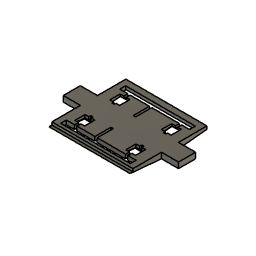
battery mount top v9 (Autodesk Fusion 360 design; units mm, degrees)
Autodesk Fusion 360 part; units mm, degrees
note: some values were not read from the file. Set by a fixed rule: which face or edge a step refers to.
sketch "Sketch1" plane through (0, 0, 0) normal (0, 0, 1) x (1, 0, 0)
  line L0 (0, 0) -> (180.975, 0)
  line L1 (0, 0) -> (0, -165.1)
  line L2 (0, -165.1) -> (180.975, -165.1)
  line L3 (180.975, 0) -> (180.975, -165.1)
  dimension "d1" = 180.975
  dimension "d2" = 180.975
  dimension "d36" = 165.1
  constraint coincident L0.start L1.start
  constraint horizontal L0
  constraint perpendicular L0 L1
  constraint perpendicular L1 L2
  measures "d1" distance of L0.start L0.end
  measures "d2" distance of L1.end L2.end
  measures "d36" distance of L0 L2
extrude "Extrude1" add sketch "Sketch1" along normal blind 6.35
sketch "Sketch2" plane through (0, 0, 6.35) normal (0, 0, 1) x (-1, 0, 0)
  line L0 (0, 0) -> (0, 165.1)
  line L1 (0, 165.1) -> (-180.975, 165.1)
  line L2 (-180.975, 165.1) -> (-180.975, 0)
  line L3 (-180.975, 0) -> (0, 0)
sketch "Sketch4" plane through (0, 0, 0) normal (0, 0, -1) x (1, 0, 0)
  line L0 (0, 165.1) -> (0, 0)
  line L1 (0, 0) -> (180.975, 0)
  line L2 (180.975, 0) -> (180.975, 165.1)
  line L3 (180.975, 165.1) -> (0, 165.1)
  line L4 (193.675, 57.15) -> (0, 57.15)
  line L5 (0, 107.95) -> (193.675, 107.95)
  line L6 (180.975, 0, -6.35) -> (0, 0, -6.35)
  line L7 (0, 165.1, -6.35) -> (180.975, 165.1, -6.35)
  line L8 (193.675, 107.95) -> (193.675, 57.15)
  dimension "d33" = 50.8
  dimension "d34" = 57.15
  dimension "d41" = 193.675
  constraint coincident L0 L4.end
  constraint perpendicular L0 L4
  constraint coincident L0 L5.start
  constraint perpendicular L2 L5
  measures "d33" distance of L4 L5
  measures "d34" distance of L1 L4
  measures "d41" distance of L5.start L5.end
sketch "Sketch5" plane through (0, 0, 0) normal (1, 0, 0) x (0, 1, 0)
  line L0 (-69.85, -6.35) -> (0, 0)
  line L1 (-95.2638, -6.3731) -> (-165.1, 0)
  line L2 (-69.85, -6.35) -> (-69.85, 0)
  line L3 (-69.85, 0) -> (0, 0)
  line L4 (-95.2638, -6.3731) -> (-95.2638, 0)
  line L5 (-95.2638, 0) -> (-165.1, 0)
  constraint coincident L0.end L3.end
  constraint vertical L2
  constraint perpendicular L2 L3
  constraint perpendicular L3 L4
  constraint perpendicular L4 L5
sketch "Sketch10" plane through (0, 0, 0) normal (-1, 0, 0) x (0, -1, 0)
  line L0 (0, 0) -> (165.1, 0)
  line L1 (165.1, 0) -> (165.1, 6.35)
  line L2 (165.1, 6.35) -> (0, 6.35)
  line L3 (0, 6.35) -> (0, 0)
  line L4 (165.1, 0) -> (69.85, 0)
  line L5 (69.85, 0) -> (69.85, -6.35)
  constraint coincident L0.end L1.start
sketch "Sketch11" plane through (0, 0, 0) normal (0, 0, -1) x (1, 0, 0)
  line L0 (0, 165.1) -> (0, 0)
  line L1 (0, 0) -> (180.975, 0)
  line L2 (180.975, 0) -> (180.975, 165.1)
  line L3 (180.975, 165.1) -> (0, 165.1)
  line L4 (-38.1, 101.6) -> (219.075, 101.6)
  line L5 (219.075, 101.6) -> (219.075, 63.5)
  line L6 (219.075, 63.5) -> (-38.1, 63.5)
  line L7 (-38.1, 63.5) -> (-38.1, 101.6)
  dimension "d67" = 38.1
  dimension "d68" = 38.1
  dimension "d69" = 38.1
  dimension "d70" = 63.5
  dimension "d71" = 165.1
  constraint horizontal L4
  constraint vertical L5
  constraint horizontal L6
  constraint vertical L7
  measures "d67" distance of L0 L7
  measures "d68" distance of L2 L5
  measures "d69" distance of L4 L6
  measures "d70" distance of L3 L4
  measures "d71" distance of L0.start L0.end
extrude "Extrude12" add sketch "Sketch11" along normal blind 6.35 and the other way blind 6.35 contours L0 L2 L4 L6 | L0 L4 L6 L7 | L2 L4 L5 L6
sketch "Sketch12" plane through (0, 0, 0) normal (1, 0, 0) x (0, 1, 0)
  line L0 (-101.6, -6.35) -> (-171.4692, 0)
  line L1 (-171.4692, 0) -> (-101.6, 0)
  line L2 (-101.6, 0) -> (-101.6, -6.35)
  line L3 (-63.5, -6.35) -> (0, 0)
  line L4 (0, 0) -> (-63.5, 0)
  line L5 (-63.5, 0) -> (-63.5, -6.35)
  line L6 (-101.6, -6.35, 219.075) -> (-101.6, -6.35, -38.1)
  line L7 (-63.5, -6.35, -38.1) -> (-63.5, -6.35, 219.075)
  point P0 (-63.5, 0)
  constraint horizontal L1
  constraint perpendicular L1 L2
  constraint coincident L3.end L4.start
  constraint perpendicular L2 L4
  constraint parallel L2 L5
  constraint coincident P0 L4.end
extrude "Extrude13" add sketch "Sketch12" along normal up to surface (180.975 mm away)
sketch "Sketch13" plane through (0, -1.4047, -15.4562) normal (0, -0.090511, -0.995895) x (1, 0, 0)
  line L0 (180.975, 100.6082) -> (180.975, 170.7654)
  line L1 (0, 170.7654) -> (0, 100.6082)
  line L2 (180.975, 170.7654) -> (0, 170.7654)
  line L3 (-89.535, 82.5409) -> (270.51, 82.5409)
  line L4 (161.925, 110.2854) -> (131.925, 110.2854)
  line L5 (131.925, 110.2854) -> (131.925, 140.2854)
  line L6 (131.925, 140.2854) -> (161.925, 140.2854)
  line L7 (161.925, 140.2854) -> (161.925, 110.2854)
  line L8 (12.7, 158.0654) -> (168.275, 158.0654)
  line L9 (168.275, 158.0654) -> (168.275, 145.3654)
  line L10 (168.275, 145.3654) -> (12.7, 145.3654)
  line L11 (12.7, 145.3654) -> (12.7, 158.0654)
  line L12 (49.05, 140.2854) -> (49.05, 110.2854)
  line L13 (19.05, 140.2854) -> (49.05, 140.2854)
  line L14 (19.05, 110.2854) -> (19.05, 140.2854)
  line L15 (49.05, 110.2854) -> (19.05, 110.2854)
  line L16 (81.4496, 145.3654) -> (76.3696, 145.3654)
  line L17 (76.3696, 145.3654) -> (76.3696, 109.8054)
  line L18 (76.3696, 109.8054) -> (81.4496, 109.8054)
  line L19 (81.4496, 109.8054) -> (81.4496, 145.3654)
  line L20 (36.2004, 145.3654) -> (31.1204, 145.3654)
  line L21 (31.1204, 145.3654) -> (31.1204, 109.8054)
  line L22 (31.1204, 109.8054) -> (36.2004, 109.8054)
  line L23 (36.2004, 109.8054) -> (36.2004, 145.3654)
  line L24 (149.9348, 145.3654) -> (144.8548, 145.3654)
  line L25 (144.8548, 145.3654) -> (144.8548, 109.8054)
  line L26 (144.8548, 109.8054) -> (149.9348, 109.8054)
  line L27 (149.9348, 109.8054) -> (149.9348, 145.3654)
  line L28 (76.3696, 114.1232) -> (76.3696, 110.1985)
  line L29 (36.2004, 110.1985) -> (36.2004, 114.1232)
  line L30 (144.8548, 136.3032) -> (144.8548, 110.1985)
  line L31 (81.4496, 110.1985) -> (81.4496, 113.8923)
  line L32 (144.8548, 113.0707) -> (144.8548, 136.3032)
  line L33 (149.9348, 113.1663) -> (149.9348, 136.2076)
  dimension "d103" = 30
  dimension "d104" = 30
  dimension "d106" = 12.7
  dimension "d108" = 12.7
  dimension "d109" = 12.7
  dimension "d110" = 12.7
  dimension "d111" = 30.48
  dimension "d112" = 19.05
  dimension "d113" = 30
  dimension "d114" = 30
  dimension "d115" = 19.05
  dimension "d116" = 30.48
  dimension "d119" = 5.08
  dimension "d120" = 35.56
  dimension "d121" = 5.08
  dimension "d122" = 35.56
  dimension "d123" = 5.08
  dimension "d124" = 35.56
  constraint horizontal L4
  constraint vertical L5
  constraint horizontal L6
  constraint vertical L7
  constraint horizontal L8
  constraint vertical L9
  constraint horizontal L10
  constraint vertical L11
  constraint horizontal L15
  constraint vertical L14
  constraint horizontal L13
  constraint vertical L12
  constraint horizontal L16
  constraint vertical L17
  constraint horizontal L18
  constraint vertical L19
  constraint coincident L10 L16.start
  constraint horizontal L20
  constraint vertical L21
  constraint horizontal L22
  constraint vertical L23
  constraint coincident L10 L20.start
  constraint horizontal L24
  constraint vertical L25
  constraint horizontal L26
  constraint vertical L27
  constraint coincident L10 L24.start
  constraint vertical L28
  constraint vertical L29
  constraint coincident L17 L28.end
  constraint coincident L23 L29.end
  constraint vertical L30
  constraint vertical L31
  constraint coincident L25 L30.end
  constraint coincident L19 L31.end
  constraint vertical L32
  constraint coincident L25 L30.start
  constraint vertical L33
  constraint coincident L27 L33.end
  measures "d103" distance of L4.start L4.end
  measures "d104" distance of L4.start L6.end
  measures "d106" distance of L8.start L10.end
  measures "d108" distance of L1 L11
  measures "d109" distance of L0 L9
  measures "d110" distance of L2 L8
  measures "d111" distance of L2 L6
  measures "d112" distance of L0 L7
  measures "d113" distance of L12.end L14.start
  measures "d114" distance of L12.start L12.end
  measures "d115" distance of L1 L14
  measures "d116" distance of L2 L13
  measures "d119" distance of L16.start L16.end
  measures "d120" distance of L16.start L18.end
  measures "d121" distance of L20.start L20.end
  measures "d122" distance of L20.start L22.end
  measures "d123" distance of L24.start L24.end
  measures "d124" distance of L24.start L26.end
sketch "Sketch14" plane through (0, 0, -6.35) normal (0, 0, -1) x (1, 0, 0)
  line L0 (-38.1, 63.5) -> (0, 63.5)
  line L1 (219.075, 63.5) -> (219.075, 101.6)
  line L2 (219.075, 101.6) -> (180.975, 101.6)
  line L3 (-38.1, 101.6) -> (-38.1, 63.5)
  line L4 (-6.35, 95.885) -> (0.127, 95.885)
  line L5 (0.127, 95.885) -> (0.127, 70.231)
  line L6 (0.127, 70.231) -> (-6.35, 70.231)
  line L7 (-6.35, 70.231) -> (-6.35, 95.885)
  line L8 (181.102, 95.885) -> (187.579, 95.885)
  line L9 (187.579, 95.885) -> (187.579, 70.231)
  line L10 (187.579, 70.231) -> (181.102, 70.231)
  line L11 (181.102, 70.231) -> (181.102, 95.885)
  line L12 (180.975, 101.6) -> (0, 101.6)
  line L13 (0, 101.6) -> (-38.1, 101.6)
  line L14 (0, 63.5) -> (180.975, 63.5)
  line L15 (180.975, 63.5) -> (219.075, 63.5)
  dimension "d80" = 25.654
  dimension "d81" = 6.477
  dimension "d82" = 5.715
  dimension "d83" = 25.654
  dimension "d84" = 6.477
  dimension "d85" = 5.715
  dimension "d87" = 180.975
  dimension "d88" = 31.75
  constraint horizontal L4
  constraint vertical L5
  constraint horizontal L6
  constraint vertical L7
  constraint horizontal L8
  constraint vertical L9
  constraint horizontal L10
  constraint vertical L11
  measures "d80" distance of L4.start L6.end
  measures "d81" distance of L4.start L4.end
  measures "d82" distance of L2 L4
  measures "d83" distance of L8.end L9.end
  measures "d84" distance of L8.start L8.end
  measures "d85" distance of L2 L8
  measures "d87" distance of L5 L11
  measures "d88" distance of L3 L7
extrude "Extrude15" cut sketch "Sketch14" against normal blind 7.62 contours L4 L5 L6 L7 | L8 L9 L10 L11
extrude "Extrude16" cut sketch "Sketch13" against normal blind 12.7 contours L4 L25 L26 L27 L30 | L4 L6 L25 L27 L30 L32 L33 | L6 L10 L24 L25 L27 | L8 L9 L10 L11 L16 L20 L24 | L10 L16 L17 L18 L19 L28 L31 | L10 L13 L20 L21 L23 | L13 L15 L21 L23 L29 | L15 L21 L22 L23 L29
extrude "Extrude17" cut sketch "Sketch13" against normal blind 5.08 contours L4 L6 L7 L27 L33 | L4 L5 L6 L25 L30 L32 | L12 L13 L15 L23 L29 | L13 L14 L15 L21
sketch "Sketch15" plane through (0, -1.4047, -15.4562) normal (0, -0.090511, -0.995895) x (1, 0, 0)
  line L0 (31.1204, 136.4754) -> (22.8654, 136.4754)
  line L1 (22.8654, 136.4754) -> (22.8654, 114.0954)
  line L2 (22.8654, 114.0954) -> (31.1204, 114.0954)
  line L3 (31.1204, 114.0954) -> (31.1204, 136.4754)
  line L4 (36.2004, 136.4754) -> (44.4554, 136.4754)
  line L5 (44.4554, 136.4754) -> (44.4554, 114.0954)
  line L6 (44.4554, 114.0954) -> (36.2004, 114.0954)
  line L7 (36.2004, 114.0954) -> (36.2004, 136.4754)
  line L8 (36.2004, 109.8054) -> (36.2004, 145.3654)
  line L9 (31.1204, 145.3654) -> (31.1204, 109.8054)
  line L10 (19.05, 140.2854) -> (49.05, 140.2854)
  line L11 (49.05, 110.2854) -> (19.05, 110.2854)
  line L12 (144.8548, 136.4754) -> (136.5998, 136.4754)
  line L13 (136.5998, 136.4754) -> (136.5998, 114.0954)
  line L14 (136.5998, 114.0954) -> (144.8548, 114.0954)
  line L15 (144.8548, 114.0954) -> (144.8548, 136.4754)
  line L16 (149.9348, 136.4754) -> (158.1898, 136.4754)
  line L17 (158.1898, 136.4754) -> (158.1898, 114.0954)
  line L18 (158.1898, 114.0954) -> (149.9348, 114.0954)
  line L19 (149.9348, 114.0954) -> (149.9348, 136.4754)
  line L20 (131.925, 140.2854) -> (161.925, 140.2854)
  line L21 (161.925, 110.2854) -> (131.925, 110.2854)
  line L22 (144.8548, 145.3654) -> (144.8548, 109.8054)
  line L23 (149.9348, 109.8054) -> (149.9348, 145.3654)
  dimension "d127" = 8.255
  dimension "d128" = 8.255
  dimension "d129" = 3.81
  dimension "d130" = 3.81
  dimension "d131" = 3.81
  dimension "d132" = 3.81
  dimension "d133" = 3.81
  dimension "d134" = 3.81
  dimension "d135" = 3.81
  dimension "d136" = 3.81
  dimension "d137" = 8.255
  dimension "d138" = 8.255
  constraint horizontal L0
  constraint vertical L1
  constraint horizontal L2
  constraint vertical L3
  constraint horizontal L4
  constraint vertical L5
  constraint horizontal L6
  constraint vertical L7
  constraint coincident L4.start L8
  constraint coincident L0.start L9
  constraint horizontal L12
  constraint vertical L13
  constraint horizontal L14
  constraint vertical L15
  constraint horizontal L16
  constraint vertical L17
  constraint horizontal L18
  constraint vertical L19
  constraint coincident L12.start L22
  constraint coincident L16.start L23
  measures "d127" distance of L0.start L0.end
  measures "d128" distance of L4.start L4.end
  measures "d129" distance of L0 L10
  measures "d130" distance of L2 L11
  measures "d131" distance of L4 L10
  measures "d132" distance of L6 L11
  measures "d133" distance of L12 L20
  measures "d134" distance of L14 L21
  measures "d135" distance of L16 L20
  measures "d136" distance of L18 L21
  measures "d137" distance of L16.start L16.end
  measures "d138" distance of L12.start L12.end
extrude "Extrude18" cut sketch "Sketch15" against normal blind 12.7 contours L0 L1 L2 L3 L9 | L4 L5 L6 L7 L8 | L12 L13 L14 L15 L22 | L16 L17 L18 L19 L23
sketch "Sketch17" plane through (0, 0, 0) normal (0, 0.099504, -0.995037) x (-1, 0, 0)
  line L0 (-180.975, 0) -> (-180.975, -63.8167)
  line L1 (0, -63.8167) -> (0, 0)
  line L2 (0, 0) -> (-180.975, 0)
  line L3 (-168.275, -25.4) -> (-12.7, -25.4)
  line L4 (-12.7, -25.4) -> (-12.7, -12.7)
  line L5 (-12.7, -12.7) -> (-168.275, -12.7)
  line L6 (-168.275, -12.7) -> (-168.275, -25.4)
  line L7 (-180.975, -63.8167) -> (0, -63.8167)
  line L8 (-35.56, -25.4) -> (-30.48, -25.4)
  line L9 (-30.48, -25.4) -> (-30.48, -60.96)
  line L10 (-30.48, -60.96) -> (-35.56, -60.96)
  line L11 (-35.56, -60.96) -> (-35.56, -25.4)
  line L12 (-83.82, -25.4) -> (-78.74, -25.4)
  line L13 (-78.74, -25.4) -> (-78.74, -60.96)
  line L14 (-78.74, -60.96) -> (-83.82, -60.96)
  line L15 (-83.82, -60.96) -> (-83.82, -25.4)
  line L16 (-145.415, -25.4) -> (-150.495, -25.4)
  line L17 (-150.495, -25.4) -> (-150.495, -60.96)
  line L18 (-150.495, -60.96) -> (-145.415, -60.96)
  line L19 (-145.415, -60.96) -> (-145.415, -25.4)
  line L20 (-47.78, -60.48) -> (-17.78, -60.48)
  line L21 (-17.78, -60.48) -> (-17.78, -30.48)
  line L22 (-17.78, -30.48) -> (-47.78, -30.48)
  line L23 (-47.78, -30.48) -> (-47.78, -60.48)
  line L24 (-133.195, -60.48) -> (-163.195, -60.48)
  line L25 (-163.195, -60.48) -> (-163.195, -30.48)
  line L26 (-163.195, -30.48) -> (-133.195, -30.48)
  line L27 (-133.195, -30.48) -> (-133.195, -60.48)
  dimension "d141" = 12.7
  dimension "d142" = 12.7
  dimension "d143" = 12.7
  dimension "d144" = 12.7
  dimension "d145" = 5.08
  dimension "d146" = 35.56
  dimension "d147" = 30.48
  dimension "d148" = 5.08
  dimension "d149" = 35.56
  dimension "d150" = 5.08
  dimension "d151" = 35.56
  dimension "d152" = 30.48
  dimension "d153" = 30
  dimension "d154" = 30
  dimension "d155" = 17.78
  dimension "d156" = 30
  dimension "d157" = 30
  dimension "d158" = 17.78
  dimension "d159" = 30.48
  dimension "d160" = 30.48
  constraint horizontal L3
  constraint vertical L4
  constraint horizontal L5
  constraint vertical L6
  constraint horizontal L8
  constraint vertical L9
  constraint horizontal L10
  constraint vertical L11
  constraint coincident L3 L8.start
  constraint horizontal L12
  constraint vertical L13
  constraint horizontal L14
  constraint vertical L15
  constraint coincident L3 L12.start
  constraint horizontal L16
  constraint vertical L17
  constraint horizontal L18
  constraint vertical L19
  constraint coincident L3 L16.start
  constraint horizontal L20
  constraint vertical L21
  constraint horizontal L22
  constraint vertical L23
  constraint horizontal L24
  constraint vertical L25
  constraint horizontal L26
  constraint vertical L27
  measures "d141" distance of L3.end L4.end
  measures "d142" distance of L1 L4
  measures "d143" distance of L0 L6
  measures "d144" distance of L2 L5
  measures "d145" distance of L9.end L10.end
  measures "d146" distance of L8.end L9.end
  measures "d147" distance of L1 L9
  measures "d148" distance of L12.start L12.end
  measures "d149" distance of L12.start L14.end
  measures "d150" distance of L16.start L16.end
  measures "d151" distance of L16.start L18.end
  measures "d152" distance of L0 L17
  measures "d153" distance of L20.start L20.end
  measures "d154" distance of L20.start L22.end
  measures "d155" distance of L1 L21
  measures "d156" distance of L24.start L24.end
  measures "d157" distance of L24.start L26.end
  measures "d158" distance of L0 L25
  measures "d159" distance of L2 L26
  measures "d160" distance of L2 L22
extrude "Extrude19" cut sketch "Sketch17" against normal blind 15.24 contours L3 L4 L5 L6 L8 L12 L16 | L3 L16 L17 L19 L26 | L17 L19 L24 L26 | L3 L12 L13 L14 L15 | L3 L8 L9 L11 L22 | L9 L11 L20 L22
extrude "Extrude20" cut sketch "Sketch17" against normal blind 5.08 contours L17 L24 L25 L26 | L19 L24 L26 L27 | L9 L20 L21 L22 | L11 L20 L22 L23
sketch "Sketch18" plane through (0, 0, 0) normal (0, 0.099504, -0.995037) x (-1, 0, 0)
  line L0 (-30.48, -56.67) -> (-22.225, -56.67)
  line L1 (-22.225, -56.67) -> (-22.225, -34.29)
  line L2 (-22.225, -34.29) -> (-30.48, -34.29)
  line L3 (-30.48, -34.29) -> (-30.48, -56.67)
  line L4 (-35.56, -56.67) -> (-43.815, -56.67)
  line L5 (-43.815, -56.67) -> (-43.815, -34.29)
  line L6 (-43.815, -34.29) -> (-35.56, -34.29)
  line L7 (-35.56, -34.29) -> (-35.56, -56.67)
  line L8 (-145.415, -56.67) -> (-137.16, -56.67)
  line L9 (-137.16, -56.67) -> (-137.16, -34.29)
  line L10 (-137.16, -34.29) -> (-145.415, -34.29)
  line L11 (-145.415, -34.29) -> (-145.415, -56.67)
  line L12 (-150.495, -56.67) -> (-158.75, -56.67)
  line L13 (-158.75, -56.67) -> (-158.75, -34.29)
  line L14 (-158.75, -34.29) -> (-150.495, -34.29)
  line L15 (-150.495, -34.29) -> (-150.495, -56.67)
  line L16 (-47.78, -60.48) -> (-17.78, -60.48)
  line L17 (-17.78, -30.48) -> (-47.78, -30.48)
  line L18 (-163.195, -30.48) -> (-133.195, -30.48)
  line L19 (-133.195, -60.48) -> (-163.195, -60.48)
  line L20 (-150.495, -25.4) -> (-150.495, -60.96)
  line L21 (-145.415, -60.96) -> (-145.415, -25.4)
  line L22 (-30.48, -25.4) -> (-30.48, -60.96)
  line L23 (-35.56, -60.96) -> (-35.56, -25.4)
  dimension "d165" = 8.255
  dimension "d166" = 8.255
  dimension "d167" = 8.255
  dimension "d168" = 8.255
  dimension "d169" = 3.81
  dimension "d170" = 3.81
  dimension "d171" = 3.81
  dimension "d172" = 3.81
  dimension "d173" = 3.81
  dimension "d174" = 3.81
  dimension "d175" = 3.81
  dimension "d176" = 3.81
  constraint horizontal L0
  constraint vertical L1
  constraint horizontal L2
  constraint vertical L3
  constraint horizontal L4
  constraint vertical L5
  constraint horizontal L6
  constraint vertical L7
  constraint horizontal L8
  constraint vertical L9
  constraint horizontal L10
  constraint vertical L11
  constraint horizontal L12
  constraint vertical L13
  constraint horizontal L14
  constraint vertical L15
  constraint coincident L12.start L20
  constraint coincident L8.start L21
  constraint coincident L0.start L22
  constraint coincident L4.start L23
  measures "d165" distance of L0.start L0.end
  measures "d166" distance of L4.start L4.end
  measures "d167" distance of L8.start L8.end
  measures "d168" distance of L12.start L12.end
  measures "d169" distance of L0 L16
  measures "d170" distance of L2 L17
  measures "d171" distance of L6 L17
  measures "d172" distance of L4 L16
  measures "d173" distance of L10 L18
  measures "d174" distance of L8 L19
  measures "d175" distance of L12 L19
  measures "d176" distance of L14 L18
extrude "Extrude21" cut sketch "Sketch18" against normal blind 15.24 contours L0 L1 L2 L3 L22 | L4 L5 L6 L7 L23 | L8 L9 L10 L11 L21 | L12 L13 L14 L15 L20
equation "d34 = 0.5 * d36 - ( ( 1 ) * 1 in )"
equation "d70 = 0.5 * d71 - 0.75 in"
equation "d83 = d80"
equation "d84 = d81"
equation "d85 = d82"
equation "d166 = d165"
equation "d167 = d165"
equation "d168 = d165"
equation "d171 = d170"
equation "d172 = d169"
equation "d173 = d169"
equation "d174 = d173"
equation "d175 = d174"
equation "d176 = d173"
